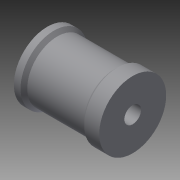
# Autodesk Inventor part: spool
Saved by Autodesk Inventor 2013 (Build 170138000, 138)
## iProperties
Created: 2014-02-26
Part Number: spool
Material: Generic
Document SubType Name: Modeling
Designer: employee
Density: 1 g/cm^3
Author: employee
Autodesk Inventor part; units mm, degrees
ref_plane "YZ Plane" through (0, 0, 0) normal (1, 0, 0) x (0, 1, 0)
ref_plane "XZ Plane" through (0, 0, 0) normal (0, 1, 0) x (-1, 0, 0)
ref_plane "XY Plane" through (0, 0, 0) normal (0, 0, 1) x (1, 0, 0)
sketch "Sketch1" plane through (0, 0, 0) normal (0, 0, 1) x (1, 0, 0)
  line L0 (0, 0) -> (25.5, 0)
  line L1 (25.5, 0) -> (25.5, 10)
  line L2 (25.5, 10) -> (21, 10)
  line L3 (21, 10) -> (20, 9)
  line L4 (20, 9) -> (3, 9)
  line L5 (3, 9) -> (2, 10)
  line L6 (2, 10) -> (0, 10)
  line L7 (0, 10) -> (0, 0)
  dimension "d0" = 25.5
  dimension "d1" = 9
  dimension "d2" = 17
  dimension "d3" = 1
  dimension "d4" = 2
  constraints: 16 end point, 4 parallel, 3 perpendicular, 1 horizontal, 1 horizontal alignment
  measures "d0" distance of L0.start L0.end
  measures "d1" distance between parallel lines of L4 L0
  measures "d2" distance of L3.end L4.end
  measures "d3" distance between parallel lines of L4 L2
  measures "d4" distance of L5.end L6.end
revolve "Revolution1" add sketch "Sketch1" angle 360 about axis through (0, 0, 0) along (1, 0, 0)
sketch "Sketch2" plane through (25.5, 0, 0) normal (1, 0, 0) x (0, 0, -1)
  circle A0 centre (0, 0) radius 10 projected
  circle A1 centre (0, 0) radius 2.5
  dimension "d6" = 5
  constraints: 1 centre point, 1 coincident
  measures "d6" diameter of A1
extrude "Extrusion1" cut sketch "Sketch2" against normal through all contours A1
body "Solid1"
